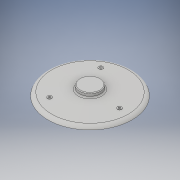
# Autodesk Inventor part: Alojamento do Sensor de Temperatura e Umidade - tampa
Saved by Autodesk Inventor 2019.4 (Build 234330000, 330)
## iProperties
Created: 2021-02-17
Part Number: Alojamento do Sensor de Temperatura e Umidade - tampa
Material: Genérico
Document SubType Name: Modeling
Designer: Lattes
Density: 1 g/cm^3
Appearance: Padrão
Author: Lattes
Autodesk Inventor part; units mm, degrees
ref_plane "YZ Plane" through (0, 0, 0) normal (1, 0, 0) x (0, 1, 0)
ref_plane "XZ Plane" through (0, 0, 0) normal (0, 1, 0) x (-1, 0, 0)
sketch "Esboço1" plane through (0, 0, 0) normal (0, 0, 1) x (1, 0, 0)
  line L0 (0, 14) -> (14, 14)
  line L1 (15, 13) -> (15, 9.830108)
  line L2 (16.82292, 7.837963) -> (54.531239, 4.486112)
  line L3 (0.6, 13.4) -> (13.4, 13.4)
  line L4 (14.4, 12.4) -> (14.4, 9.281076)
  line L5 (16.22292, 7.28893) -> (53.931239, 3.93708)
  line L6 (0.6, 13.4) -> (0, 13.4)
  line L7 (0, 14) -> (0, 13.4)
  line L8 (0, 0) -> (0, 5.450968)
  arc A0 (59.042785, 0) -> (53.931239, 3.93708) centre (53.4, -2.039356) ccw
  arc A1 (59.811965, 0) -> (54.531239, 4.486112) centre (54, -1.490324) ccw
  line L9 (59.811965, 0) -> (59.042785, 0)
  arc A2 (15, 9.830108) -> (16.82292, 7.837963) centre (17, 9.830108) ccw
  arc A3 (14.4, 9.281076) -> (16.22292, 7.28893) centre (16.4, 9.281076) ccw
  arc A4 (14.4, 12.4) -> (13.4, 13.4) centre (13.4, 12.4) ccw
  arc A5 (15, 13) -> (14, 14) centre (14, 13) ccw
  point P0 (60, 4)
  point P1 (15, 14)
  point P2 (15, 8)
  dimension "d4" = 15
  dimension "d5" = 6
  dimension "d7" = 6
  dimension "d8" = 2
  dimension "d9" = 1
  constraints: 20 end point, 12 point on circle, 10 tangent, 6 centre point, 6 point on line, 3 equal radius, 2 horizontal, 2 perpendicular, 1 vertical, 2 other
  measures "d4" distance of L0.start point (15, 14)
  measures "d5" distance of point (15, 14) point (15, 8)
  measures "d7" radius of A0
  measures "d8" radius of A2
  measures "d9" radius of A4
sketch "Esboço1 outline for Revolução1" plane through (0, 0, 0) normal (0, 0, 1) x (1, 0, 0)
  line L0 (0, 14) -> (14, 14)
  arc A0 (14, 14) -> (15, 13) centre (14, 13) cw
  line L1 (15, 13) -> (15, 9.830108)
  arc A1 (15, 9.830108) -> (16.82292, 7.837963) centre (17, 9.830108) ccw
  line L2 (16.82292, 7.837963) -> (54.531239, 4.486112)
  arc A2 (54.531239, 4.486112) -> (59.811965, 0) centre (54, -1.490324) cw
  line L3 (59.811965, 0) -> (59.042785, 0)
  arc A3 (59.042785, 0) -> (53.931239, 3.93708) centre (53.4, -2.039356) ccw
  line L4 (53.931239, 3.93708) -> (16.22292, 7.28893)
  arc A4 (16.22292, 7.28893) -> (14.4, 9.281076) centre (16.4, 9.281076) cw
  line L5 (14.4, 9.281076) -> (14.4, 12.4)
  arc A5 (14.4, 12.4) -> (13.4, 13.4) centre (13.4, 12.4) ccw
  line L6 (13.4, 13.4) -> (0.6, 13.4)
  line L7 (0.6, 13.4) -> (0, 13.4)
  line L8 (0, 13.4) -> (0, 14)
revolve "Revolução1" add sketch "Esboço1 outline for Revolução1" angle 360 about axis through (0, 0, 0) along (0, 1, 0)
sketch "Esboço2" plane through (0, 14, 0) normal (0, 1, 0) x (1, 0, 0)
  line L0 (0, 0) -> (42, 0)
  circle A0 centre (42, 0) radius 1.5
  dimension "d11" = 42
  dimension "d12" = 3
  constraints: 2 end point, 1 centre point, 1 coincident, 1 horizontal
  measures "d11" distance of L0.start L0.end
  measures "d12" diameter of A0
sketch "Esboço2 outline for Extrusão1" plane through (0, 14, 0) normal (0, 1, 0) x (1, 0, 0)
  circle A0 centre (42, 0) radius 1.5
extrude "Extrusão1" cut sketch "Esboço2 outline for Extrusão1" against normal blind 20
pattern_circular "Padrão circular1" count 3 over 360 about axis through (0, 6.162037, 0) along (0, -1, 0) of "Extrusão1"
ref_plane "Plano de trabalho1" through (0, 6, 0) normal (0, 1, 0) x (1, 0, 0)
sketch "Esboço4" plane through (0, 6, 0) normal (0, 1, 0) x (1, 0, 0)
  line L0 (0, 0) -> (42, 0)
  circle A0 centre (42, 0) radius 1.5
  circle A1 centre (42, 0) radius 3
  dimension "d21" = 42
  dimension "d22" = 3
  dimension "d23" = 6
  constraints: 2 centre point, 2 coincident, 2 end point, 1 horizontal
  measures "d21" distance of L0.start L0.end
  measures "d22" diameter of A0
  measures "d23" diameter of A1
sketch "Esboço4 outline for Extrusão2" plane through (0, 6, 0) normal (0, 1, 0) x (1, 0, 0)
  circle A0 centre (42, 0) radius 3
  circle A1 centre (42, 0) radius 1.5
extrude "Extrusão2" add sketch "Esboço4 outline for Extrusão2" against normal blind 3
pattern_circular "Padrão circular2" count 3 over 360 about axis through (0, 5.613005, 0) along (0, -1, 0) of "Extrusão2"
